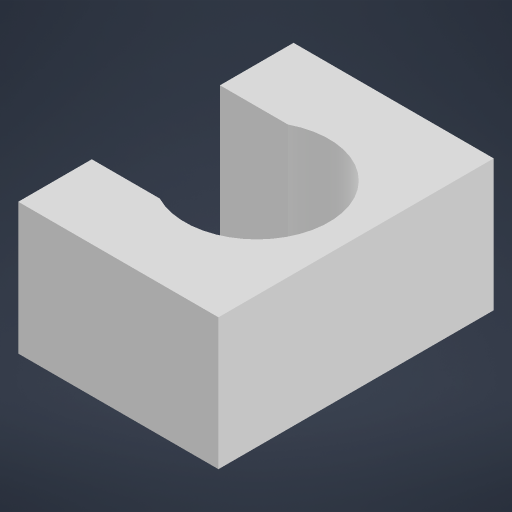
# Autodesk Inventor part: WireSlot
Saved by Autodesk Inventor 2024.1 (Build 281209000, 209)
## iProperties
Created: 2023-08-17
Part Number: WireSlot
Material: Generic
Document SubType Name: Modeling
Designer: Eleanor
Density: 1 g/cm^3
Appearance: Default
Mass: 0.00112987 g
Surface Area: 0.0934343 cm^2
Volume: 0.00112987 cm^3
Author: Eleanor
Autodesk Inventor part; units mm, degrees
ref_plane "YZ Plane" through (0, 0, 0) normal (1, 0, 0) x (0, 1, 0)
ref_plane "XZ Plane" through (0, 0, 0) normal (0, 1, 0) x (-1, 0, 0)
ref_plane "XY Plane" through (0, 0, 0) normal (0, 0, 1) x (1, 0, 0)
sketch "Sketch1" plane through (0, 0, 2.1048) normal (1, 0, 0) x (0, 1, 0)
  line L0 (-5.8691, -5.0828) -> (5.8691, -5.0828)
  line L1 (-3.9283, -0.8731) -> (-3.9283, 0.8731)
  line L2 (-3.9283, 0.8731) -> (-4.7625, 0.8731)
  line L3 (-4.7625, 0.8731) -> (-4.7625, -0.8731)
  line L4 (-4.7625, -0.8731) -> (-3.9283, -0.8731)
  line L5 (-3.9283, -0.8731) -> (-4.7625, 0.8731) construction
  line L6 (-3.9283, 0.8731) -> (-4.7625, -0.8731) construction
  point P0 (0, 0)
  point P1 (1.6165, -2.7999)
  point P2 (-4.3454, 0)
  constraints: 14 end point, 2 midpoint, 2 parallel, 1 perpendicular, 1 vertical
extrude "Extrusion1" add sketch "Sketch1" along normal blind 1.27
sketch "Sketch2" plane through (-4.7625, -4.7625, 0) normal (0, -1, 0) x (-1, 0, 0)
  arc A0 (-5.1935, -1.6984) -> (-5.1935, -2.5112) centre (-5.403, -2.1048) ccw
  line L0 (-6.0325, -1.2317) -> (-12.065, -1.2317)
  line L1 (-4.7625, -2.9779) -> (-6.0325, -2.9779) projected
  arc A1 (-5.1935, -1.6984) -> (-5.1935, -2.5112) centre (-5.403, -2.1048) ccw
  line L2 (-6.0325, -2.9779) -> (-6.0325, -1.2317) projected
  line L3 (-5.1935, -1.6984) -> (-4.7277, -1.6984)
  line L4 (-4.7277, -2.5112) -> (-5.1935, -2.5112)
  line L5 (-4.7277, -1.6984) -> (-4.7277, -2.5112)
  point P0 (-3.175, 0.8731)
  point P1 (0, 1.7462)
  point P2 (0, 0)
  point P3 (-6.0325, -2.1048)
  point P4 (-4.997, -2.5282)
  point P5 (-5.0204, -1.6646)
  dimension "d11" = 0.8731
  dimension "d13" = 0.4572
  dimension "d14" = 0.6295
  dimension "d15" = 0.8128
  dimension "d17" = 0.4658
  dimension "d18" = 0.4658
  constraints: 8 end point, 4 point on circle, 2 centre point, 2 horizontal, 1 concentric, 1 parallel, 1 vertical
  measures "d11" distance from line of L1 A0.centre
  measures "d13" radius of A0
  measures "d14" distance from line of L2 A0.centre
  measures "d15" distance of L4.end L3.start
  measures "d17" distance of L3.start L3.end
  measures "d18" distance of L4.start L4.end
extrude "Extrusion2" cut sketch "Sketch2" against normal blind 1.27
equation "\"d18\" = d17"
body "Solid1"
